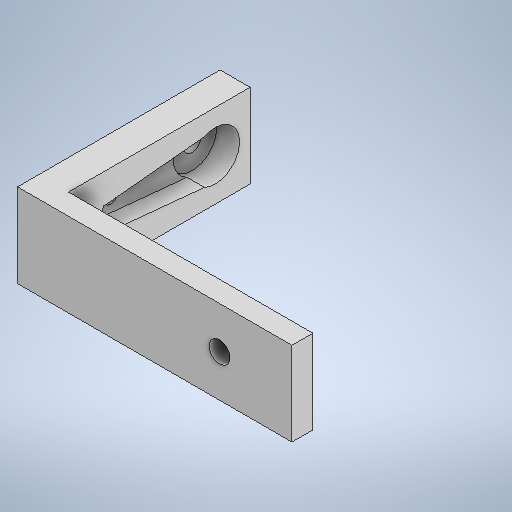
# Autodesk Inventor part: 18_2
Saved by Autodesk Inventor 2026.1 (Build 301233020, 233B)
## iProperties
Created: 2026-04-11
Part Number: 18_2
Material: Generic
Document SubType Name: Modeling
Designer: irach
Density: 1 g/cm^3
Appearance: Default
Author: irach
Autodesk Inventor part; units mm, degrees
ref_plane "YZ Plane" through (0, 0, 0) normal (1, 0, 0) x (0, 1, 0)
ref_plane "XZ Plane" through (0, 0, 0) normal (0, 1, 0) x (-1, 0, 0)
ref_plane "XY Plane" through (0, 0, 0) normal (0, 0, 1) x (1, 0, 0)
sketch "Sketch1" plane through (0, 0, 0) normal (1, 0, 0) x (0, 1, 0)
  line L0 (6.1324, -14.2794) -> (-5.8676, -14.2794)
  line L1 (-5.8676, -14.2794) -> (-5.8676, -43.2794)
  line L2 (-5.8676, -43.2794) -> (6.1324, -43.2794)
  line L3 (6.1324, -43.2794) -> (6.1324, -14.2794)
  point P0 (0, 0)
  dimension "d0" = 12
  dimension "d1" = 29
  constraints: 8 end point, 2 parallel, 1 horizontal, 1 perpendicular
  measures "d0" distance of L1.end L2.end
  measures "d1" distance of L2.end L0.start
extrude "Extrusion1" add sketch "Sketch1" along normal blind 1.8
sketch "Sketch2" plane through (1.8, 0, 0) normal (1, 0, 0) x (0, 0, -1)
  circle A0 centre (38.2794, 0.1324) radius 3.5
  line L0 (43.2794, -5.8676) -> (43.2794, 6.1324) projected
  line L1 (14.2794, -5.8676) -> (43.2794, -5.8676) projected
  point P0 (0, 0)
  dimension "d4" = 7
  dimension "d5" = 5
  dimension "d6" = 6
  constraints: 1 centre point
  measures "d4" diameter of A0
  measures "d5" distance from line of L0 A0.centre
  measures "d6" distance from line of L1 A0.centre
extrude "Extrusion2" cut sketch "Sketch2" against normal blind 0.8
sketch "Sketch3" plane through (1.8, 0, 0) normal (1, 0, 0) x (0, 0, -1)
  line L0 (14.2794, 6.1324) -> (14.2794, -5.8676) projected
  line L1 (43.2794, -5.8676) -> (43.2794, 6.1324) projected
  line L2 (14.2794, 6.1324) -> (43.2794, 6.1324)
  line L3 (43.2794, 6.1324) -> (43.2794, -5.8676)
  line L4 (43.2794, -5.8676) -> (14.2794, -5.8676)
  line L5 (14.2794, -5.8676) -> (14.2794, 6.1324)
  circle A0 centre (38.2794, 0.1324) radius 3.5 projected
  circle A1 centre (38.2794, 0.1324) radius 3.5
  point P0 (0, 0)
  point P1 (43.2794, 6.1324)
  point P2 (14.2794, -5.8676)
  constraints: 8 end point, 2 parallel, 1 centre point, 1 coincident, 1 horizontal, 1 perpendicular
extrude "Extrusion3" add sketch "Sketch3" along normal blind 2.5
sketch "Sketch4" plane through (4.3, 0, 0) normal (1, 0, 0) x (0, 0, -1)
  circle A0 centre (38.2794, 0.1324) radius 3.5 projected
  line L0 (36.7494, 3.2802) -> (22.3405, 1.8824)
  line L1 (36.7494, -3.0155) -> (22.3405, -1.6176)
  arc A1 (22.3405, 1.8824) -> (22.3405, -1.6176) centre (24.7889, 0.1324) ccw
  line L2 (43.2794, 6.1324) -> (14.2794, 6.1324) projected
  point P0 (0, 0)
  point P1 (21.7794, 0.1324)
  dimension "d15" = 1.53
  dimension "d16" = 1.53
  dimension "d17" = 16.5
  dimension "d18" = 3.5
  dimension "d19" = 6
  constraints: 5 point on circle, 4 end point, 1 centre point
  measures "d15" horizontal distance of A0.centre L0.start
  measures "d16" horizontal distance of A0.centre L1.start
  measures "d17" distance of A0.centre point (21.779, 0.132)
  measures "d18" distance of L1.end L0.end
  measures "d19" distance from line of L2 A1.centre
extrude "Extrusion4" cut sketch "Sketch4" against normal blind 2.5 contours A0 L1 A1 L0
sketch "Sketch5" plane through (0, 0, 0) normal (-1, 0, 0) x (0, 0, 1)
  circle A0 centre (-38.2794, 0.1324) radius 3.5 projected
  circle A1 centre (-38.2794, 0.1324) radius 1.25
  point P0 (0, 0)
  dimension "d22" = 2.5
  constraints: 1 centre point, 1 coincident
  measures "d22" diameter of A1
extrude "Extrusion5" cut sketch "Sketch5" against normal blind 2.5 contours A1
sketch "Sketch6" plane through (4.3, 0, 0) normal (1, 0, 0) x (0, 0, -1)
  line L0 (43.2794, 6.1324) -> (14.2794, 6.1324) projected
  line L1 (14.2794, -5.8676) -> (43.2794, -5.8676) projected
  line L2 (14.2794, 6.1324) -> (17.2794, 6.1324)
  line L3 (17.2794, 6.1324) -> (17.2794, -5.8676)
  line L4 (17.2794, -5.8676) -> (14.2794, -5.8676)
  line L5 (14.2794, -5.8676) -> (14.2794, 6.1324)
  point P0 (0, 0)
  point P1 (14.2794, -5.8676)
  point P2 (17.2794, 6.1324)
  dimension "d25" = 3
  constraints: 8 end point, 2 parallel, 1 horizontal, 1 perpendicular, 1 point on line
  measures "d25" distance of L3.end L4.end
extrude "Extrusion6" add sketch "Sketch6" along normal blind 35
sketch "Sketch7" plane through (0, -5.8676, -14.2794) normal (0, 0, 1) x (1, 0, 0)
  circle A0 centre (28.925, 6) radius 1.5
  line L0 (39.3, 12) -> (39.3, 0) projected
  line L1 (0, 12) -> (39.3, 12) projected
  line L2 (0, 12) -> (0, 0) projected
  point P0 (0, 5.8676)
  dimension "d28" = 3
  dimension "d30" = 6
  dimension "d38" = 28.925
  constraints: 1 centre point
  measures "d28" diameter of A0
  measures "d30" distance from line of A0.centre L1
  measures "d38" distance from line of A0.centre L2
extrude "Extrusion7" cut sketch "Sketch7" against normal blind 40
sketch "Sketch8" plane through (1.8, 0, 0) normal (1, 0, 0) x (0, 0, -1)
  circle A0 centre (25.7794, 0.1324) radius 1
  circle A1 centre (38.2794, 0.1324) radius 1.25 projected
  point P0 (0, 0)
  dimension "d33" = 2
  dimension "d34" = 12.5
  dimension "d35" = 0
  constraints: 1 centre point
  measures "d33" diameter of A0
  measures "d34" distance of A1.centre A0.centre
  measures "d35" vertical distance of A0.centre A1.centre
extrude "Extrusion8" cut sketch "Sketch8" against normal blind 10 contours A0
body "Solid1"
